Autodesk Fusion 360 part; units mm, degrees
note: some values were not read from the file. Set by a fixed rule: which sketch regions a step uses.
(part 2 of 4)
  dimension "d679" = 4.2
  dimension "d680" = 50.8
  dimension "d681" = 177.3195
  dimension "d682" = 177.3195
  dimension "d683" = 177.3195
  dimension "d684" = 177.3195
  dimension "d685" = 25.4
  dimension "d686" = 25.4
  dimension "d687" = 25.4
  dimension "d688" = 25.4
  dimension "d689" = 4.2
  dimension "d690" = 4.2
  dimension "d691" = 4.2
  dimension "d692" = 4.2
  dimension "d693" = 50.8
  dimension "d697" = 177.3195
  dimension "d698" = 177.3195
  dimension "d699" = 177.3195
  dimension "d700" = 177.3195
  dimension "d701" = 25.4
  dimension "d702" = 25.4
  dimension "d703" = 25.4
  dimension "d704" = 25.4
  dimension "d705" = 4.2
  dimension "d706" = 4.2
  dimension "d707" = 4.2
  dimension "d708" = 4.2
  dimension "d709" = 50.8
  dimension "d710" = 177.3195
  dimension "d711" = 177.3195
  dimension "d712" = 177.3195
  dimension "d713" = 177.3195
  dimension "d714" = 25.4
  dimension "d715" = 25.4
  dimension "d716" = 25.4
  dimension "d717" = 25.4
  dimension "d718" = 4.2
  dimension "d719" = 4.2
  dimension "d720" = 4.2
  dimension "d721" = 4.2
  dimension "d722" = 50.8
  dimension "d723" = 177.3195
  dimension "d724" = 177.3195
  dimension "d725" = 177.3195
  dimension "d726" = 177.3195
  dimension "d727" = 25.4
  dimension "d728" = 25.4
  dimension "d729" = 25.4
  dimension "d730" = 25.4
  dimension "d731" = 4.2
  dimension "d732" = 4.2
  dimension "d733" = 4.2
  dimension "d734" = 4.2
  dimension "d735" = 50.8
  constraint horizontal L6
  constraint vertical L7
  constraint horizontal L5
  constraint vertical L8
  constraint horizontal L0
  constraint perpendicular L0 L27
  constraint horizontal L19
  constraint perpendicular L2 L20
  constraint horizontal L14
  constraint perpendicular L13 L23
  constraint horizontal L4
  constraint perpendicular L29 L30
  constraint perpendicular L0 L12
  constraint tangent A9 L29
  constraint tangent A9 L27
  constraint coincident P14 L0
  constraint coincident P14 L27
  constraint tangent L0 A7
  constraint tangent A7 L27
  constraint tangent L0 A18
  constraint tangent L2 A18
  constraint coincident P13 L2
  constraint coincident P13 L20
  constraint tangent L2 A12
  constraint tangent L20 A12
  constraint coincident P7 L3
  constraint coincident P7 L12
  constraint tangent L3 A15
  constraint tangent L12 A15
  constraint coincident P11 L24
  constraint coincident P11 L12
  constraint tangent L24 A14
  constraint tangent L12 A14
  constraint coincident L14.start L20
  constraint coincident L14.start L24
  constraint tangent L20 A20
  constraint tangent L24 A20
  constraint coincident P8 L30
  constraint coincident P8 L29
  constraint tangent A10 L30
  constraint tangent A10 L29
  constraint coincident L4.start L13
  constraint coincident L4.start L30
  constraint tangent A0 L13
  constraint tangent A0 L30
  constraint coincident P12 L13
  constraint coincident P12 L23
  constraint tangent L13 A17
  constraint tangent L23 A17
  constraint coincident P6 L23
  constraint coincident P6 L3
  constraint tangent A4 L23
  constraint tangent L3 A4
  constraint horizontal L10
  constraint perpendicular L10 L21
  constraint perpendicular L11 L22
  constraint horizontal L16
  constraint perpendicular L25 L26
  constraint perpendicular L9 L17
  constraint perpendicular L10 L18
  constraint tangent L9 A19
  constraint tangent L21 A19
  constraint coincident P14 L10
  constraint coincident P14 L21
  constraint tangent L10 A3
  constraint tangent A3 L21
  constraint tangent L10 A8
  constraint tangent L11 A8
  constraint coincident P13 L11
  constraint coincident P13 L22
  constraint tangent L11 A16
  constraint tangent L22 A16
  constraint coincident P7 L28
  constraint coincident P7 L18
  constraint tangent A22 L28
  constraint tangent L18 A22
  constraint coincident P11 L15
  constraint coincident P11 L18
  constraint tangent L15 A23
  constraint tangent L18 A23
  constraint coincident L14.start L22
  constraint coincident L14.start L15
  constraint tangent A1 L22
  constraint tangent A1 L15
  constraint coincident P8 L17
  constraint coincident P8 L9
  constraint tangent A2 L17
  constraint tangent L9 A2
  constraint tangent A11 L25
  constraint tangent L17 A11
  constraint coincident P12 L25
  constraint coincident P12 L26
  constraint tangent A5 L25
  constraint tangent A5 L26
  constraint coincident P6 L26
  constraint coincident P6 L28
  constraint tangent A13 L26
  constraint tangent A13 L28
  constraint horizontal L1
  constraint coincident L1.start L0
  constraint horizontal L53
  constraint horizontal L36
  constraint horizontal L70
  constraint coincident L48.end L36
  constraint parallel L49 L53
  constraint parallel L38 L71
  constraint collinear L47 L53
  constraint collinear L36 L61
  constraint horizontal L77
  constraint horizontal L76
  constraint horizontal L59
  constraint coincident L54.end L76
  constraint parallel L67 L77
  constraint parallel L55 L64
  constraint collinear L32 L77
  constraint collinear L58 L76
  constraint perpendicular L38 L57
  constraint perpendicular L37 L71
  constraint collinear L44 L71
  constraint collinear L34 L74
  constraint perpendicular L46 L51
  constraint coincident A26.start A31
  constraint perpendicular L39 L66
  constraint concentric A26 A31
  constraint vertical L35
  constraint perpendicular L35 L41
  constraint perpendicular L31 L35
  constraint perpendicular L41 L73
  constraint coincident L65.end L41
  constraint parallel L40 L41
  constraint parallel L33 L73
  constraint parallel L31 L50
  constraint parallel L35 L75
  constraint coincident L40.end A27.centre
  constraint coincident L33.end A25.centre
  constraint coincident A29.centre L50.end
  constraint coincident A24.centre L75.end
  constraint parallel L41 L45
  constraint coincident L31.start L35.start
  constraint coincident L45.end A28
  constraint horizontal L93
  constraint vertical L96
  constraint horizontal L98
  constraint vertical L85
  constraint coincident P15 L85.end
  constraint horizontal L86
  constraint vertical L101
  constraint horizontal L87
  constraint vertical L92
  constraint coincident L87.start A32.centre
  constraint perpendicular L98 L100
  constraint vertical L83
  constraint horizontal L80
  constraint vertical L81
  constraint horizontal L82
  constraint vertical L84
  constraint horizontal L99
  constraint vertical L89
  constraint horizontal L97
  constraint vertical L95
  constraint horizontal L94
  constraint vertical L91
  constraint horizontal L88
  constraint vertical L90
  constraint coincident L89.end L97.start
  constraint coincident L88.start L91.end
  constraint horizontal L102
  constraint vertical L103
  constraint horizontal L104
  constraint vertical L105
  constraint horizontal L112
  constraint perpendicular L112 L125
  constraint horizontal L131
  constraint perpendicular L113 L119
  constraint horizontal L130
  constraint perpendicular L107 L108
  constraint horizontal L128
  constraint perpendicular L106 L116
  constraint perpendicular L112 L120
  constraint tangent L116 A42
  constraint tangent A42 L125
  constraint coincident P26 L112
  constraint coincident P26 L125
  constraint tangent L112 A52
  constraint tangent L125 A52
  constraint tangent A35 L112
  constraint tangent A35 L113
  constraint coincident P28 L113
  constraint coincident P28 L119
  constraint tangent L113 A53
  constraint tangent L119 A53
  constraint coincident P30 L109
  constraint coincident P30 L120
  constraint tangent L109 A49
  constraint tangent L120 A49
  constraint coincident P21 L118
  constraint coincident P21 L120
  constraint tangent L118 A43
  constraint tangent A43 L120
  constraint coincident L122.start L119
  constraint coincident L122.start L118
  constraint tangent L119 A51
  constraint tangent L118 A51
  constraint coincident P22 L106
  constraint coincident P22 L116
  constraint tangent L106 A37
  constraint tangent A37 L116
  constraint coincident L128.start L107
  constraint coincident L128.start L106
  constraint tangent L107 A57
  constraint tangent L106 A57
  constraint coincident P25 L107
  constraint coincident P25 L108
  constraint tangent L107 A41
  constraint tangent L108 A41
  constraint coincident P29 L108
  constraint coincident P29 L109
  constraint tangent L108 A39
  constraint tangent L109 A39
  constraint horizontal L115
  constraint perpendicular L115 L121
  constraint perpendicular L124 L132
  constraint horizontal L122
  constraint perpendicular L114 L129
  constraint perpendicular L110 L127
  constraint perpendicular L115 L123
  constraint tangent L110 A54
  constraint tangent L121 A54
  constraint coincident P26 L115
  constraint coincident P26 L121
  constraint tangent L115 A47
  constraint tangent L121 A47
  constraint tangent L115 A55
  constraint tangent A55 L132
  constraint coincident P28 L132
  constraint coincident P28 L124
  constraint tangent A40 L132
  constraint tangent A40 L124
  constraint coincident P30 L117
  constraint coincident P30 L123
  constraint tangent L117 A45
  constraint tangent A45 L123
  constraint coincident P21 L126
  constraint coincident P21 L123
  constraint tangent A50 L126
  constraint tangent A50 L123
  constraint coincident L122.start L124
  constraint coincident L122.start L126
  constraint tangent A48 L124
  constraint tangent A48 L126
  constraint coincident P22 L127
  constraint coincident P22 L110
  constraint tangent A46 L127
  constraint tangent L110 A46
  constraint tangent A36 L129
  constraint tangent A36 L127
  constraint coincident P25 L129
  constraint coincident P25 L114
  constraint tangent L129 A56
  constraint tangent L114 A56
  constraint coincident P29 L114
  constraint coincident P29 L117
  constraint tangent A38 L114
  constraint tangent A38 L117
  constraint horizontal L111
  constraint coincident L111.start L112
  constraint horizontal L139
  constraint perpendicular L139 L152
  constraint horizontal L158
  constraint perpendicular L140 L146
  constraint horizontal L157
  constraint perpendicular L134 L135
  constraint horizontal L155
  constraint perpendicular L133 L143
  constraint perpendicular L139 L147
  constraint tangent L143 A66
  constraint tangent A66 L152
  constraint coincident P41 L139
  constraint coincident P41 L152
  constraint tangent L139 A76
  constraint tangent L152 A76
  constraint tangent A59 L139
  constraint tangent A59 L140
  constraint coincident P43 L140
  constraint coincident P43 L146
  constraint tangent L140 A77
  constraint tangent L146 A77
  constraint coincident P45 L136
  constraint coincident P45 L147
  constraint tangent L136 A73
  constraint tangent L147 A73
  constraint coincident P36 L145
  constraint coincident P36 L147
  constraint tangent L145 A67
  constraint tangent A67 L147
  constraint coincident L149.start L146
  constraint coincident L149.start L145
  constraint tangent L146 A75
  constraint tangent L145 A75
  constraint coincident P37 L133
  constraint coincident P37 L143
  constraint tangent L133 A61
  constraint tangent A61 L143
  constraint coincident L155.start L134
  constraint coincident L155.start L133
  constraint tangent L134 A81
  constraint tangent L133 A81
  constraint coincident P40 L134
  constraint coincident P40 L135
  constraint tangent L134 A65
  constraint tangent L135 A65
  constraint coincident P44 L135
  constraint coincident P44 L136
  constraint tangent L135 A63
  constraint tangent L136 A63
  constraint horizontal L142
  constraint perpendicular L142 L148
  constraint perpendicular L151 L159
  constraint horizontal L149
  constraint perpendicular L141 L156
  constraint perpendicular L137 L154
  constraint perpendicular L142 L150
  constraint tangent L137 A78
  constraint tangent L148 A78
  constraint coincident P41 L142
  constraint coincident P41 L148
  constraint tangent L142 A71
  constraint tangent L148 A71
  constraint tangent L142 A79
  constraint tangent A79 L159
  constraint coincident P43 L159
  constraint coincident P43 L151
  constraint tangent A64 L159
  constraint tangent A64 L151
  constraint coincident P45 L144
  constraint coincident P45 L150
  constraint tangent L144 A69
  constraint tangent A69 L150
  constraint coincident P36 L153
  constraint coincident P36 L150
  constraint tangent A74 L153
  constraint tangent A74 L150
  constraint coincident L149.start L151
  constraint coincident L149.start L153
  constraint tangent A72 L151
  constraint tangent A72 L153
  constraint coincident P37 L154
  constraint coincident P37 L137
  constraint tangent A70 L154
  constraint tangent L137 A70
  constraint tangent A60 L156
  constraint tangent A60 L154
  constraint coincident P40 L156
  constraint coincident P40 L141
  constraint tangent L156 A80
  constraint tangent L141 A80
  constraint coincident P44 L141
  constraint coincident P44 L144
  constraint tangent A62 L141
  constraint tangent A62 L144
  constraint horizontal L138
  constraint coincident L138.start L139
  constraint horizontal L166
  constraint perpendicular L166 L179
  constraint horizontal L185
  constraint perpendicular L167 L173
  constraint horizontal L184
  constraint perpendicular L161 L162
  constraint horizontal L182
  constraint perpendicular L160 L170
  constraint perpendicular L166 L174
  constraint tangent L170 A90
  constraint tangent A90 L179
  constraint coincident P56 L166
  constraint coincident P56 L179
  constraint tangent L166 A100
  constraint tangent L179 A100
  constraint tangent A83 L166
  constraint tangent A83 L167
  constraint coincident P58 L167
  constraint coincident P58 L173
  constraint tangent L167 A101
  constraint tangent L173 A101
  constraint coincident P60 L163
  constraint coincident P60 L174
  constraint tangent L163 A97
  constraint tangent L174 A97
  constraint coincident P51 L172
  constraint coincident P51 L174
  constraint tangent L172 A91
  constraint tangent A91 L174
  constraint coincident L176.start L173
  constraint coincident L176.start L172
  constraint tangent L173 A99
  constraint tangent L172 A99
  constraint coincident P52 L160
  constraint coincident P52 L170
  constraint tangent L160 A85
  constraint tangent A85 L170
  constraint coincident L182.start L161
  constraint coincident L182.start L160
  constraint tangent L161 A105
  constraint tangent L160 A105
  constraint coincident P55 L161
  constraint coincident P55 L162
  constraint tangent L161 A89
  constraint tangent L162 A89
  constraint coincident P59 L162
  constraint coincident P59 L163
  constraint tangent L162 A87
  constraint tangent L163 A87
  constraint horizontal L169
  constraint perpendicular L169 L175
  constraint perpendicular L178 L186
  constraint horizontal L176
  constraint perpendicular L168 L183
  constraint perpendicular L164 L181
  constraint perpendicular L169 L177
  constraint tangent L164 A102
  constraint tangent L175 A102
  constraint coincident P56 L169
  constraint coincident P56 L175
  constraint tangent L169 A95
  constraint tangent L175 A95
  constraint tangent L169 A103
  constraint tangent A103 L186
  constraint coincident P58 L186
  constraint coincident P58 L178
  constraint tangent A88 L186
  constraint tangent A88 L178
  constraint coincident P60 L171
  constraint coincident P60 L177
  constraint tangent L171 A93
  constraint tangent A93 L177
  constraint coincident P51 L180
  constraint coincident P51 L177
  constraint tangent A98 L180
  constraint tangent A98 L177
  constraint coincident L176.start L178
  constraint coincident L176.start L180
  constraint tangent A96 L178
  constraint tangent A96 L180
  constraint coincident P52 L181
  constraint coincident P52 L164
  constraint tangent A94 L181
  constraint tangent L164 A94
  constraint tangent A84 L183
  constraint tangent A84 L181
  constraint coincident P55 L183
  constraint coincident P55 L168
  constraint tangent L183 A104
  constraint tangent L168 A104
  constraint coincident P59 L168
  constraint coincident P59 L171
  constraint tangent A86 L168
  constraint tangent A86 L171
  constraint horizontal L165
  constraint coincident L165.start L166
  constraint horizontal L188
  constraint vertical L190
  constraint horizontal L187
  constraint vertical L189
  constraint horizontal L205
  constraint vertical L210
  constraint horizontal L207
  constraint vertical L196
  constraint coincident P61 L195.start
  constraint horizontal L195
  constraint vertical L193
  constraint horizontal L203
  constraint vertical L206
  constraint coincident L193.end L203.start
  constraint perpendicular L198 L207
  constraint vertical L209
  constraint horizontal L192
  constraint vertical L199
  constraint horizontal L201
  constraint vertical L204
  constraint horizontal L212
  constraint vertical L211
  constraint horizontal L200
  constraint vertical L197
  constraint horizontal L194
  constraint vertical L191
  constraint horizontal L202
  constraint vertical L208
  constraint coincident L200.start A108.centre
  constraint coincident L191.end A107.centre
  constraint horizontal L227
  constraint vertical L232
  constraint horizontal L229
  constraint vertical L218
  constraint coincident P62 L217.start
  constraint horizontal L217
  constraint vertical L215
  constraint horizontal L225
  constraint vertical L228
  constraint coincident L215.end L225.start
  constraint perpendicular L220 L229
  constraint vertical L231
  constraint horizontal L214
  constraint vertical L221
  constraint horizontal L223
  constraint vertical L226
  constraint horizontal L234
  constraint vertical L233
  constraint horizontal L222
  constraint vertical L219
  constraint horizontal L216
  constraint vertical L213
  constraint horizontal L224
  constraint vertical L230
  constraint coincident L222.start A111.centre
  constraint coincident L213.end A110.centre
  constraint horizontal L249
  constraint vertical L254
  constraint horizontal L251
  constraint vertical L240
  constraint coincident P63 L239.start
  constraint horizontal L239
  constraint vertical L237
  constraint horizontal L247
  constraint vertical L250
  constraint coincident L237.end L247.start
  constraint perpendicular L242 L251
  constraint vertical L253
  constraint horizontal L236
  constraint vertical L243
  constraint horizontal L245
  constraint vertical L248
  constraint horizontal L256
  constraint vertical L255
  constraint horizontal L244
  constraint vertical L241
  constraint horizontal L238
  constraint vertical L235
  constraint horizontal L246
  constraint vertical L252
  constraint coincident L244.start A114.centre
  constraint coincident L235.end A113.centre
  constraint horizontal L261
  constraint vertical L262
  constraint horizontal L263
  constraint vertical L264
  constraint horizontal L268
  constraint vertical L266
  constraint horizontal L265
  constraint vertical L267
  constraint horizontal L273
  constraint horizontal L283
  constraint horizontal L286
  constraint coincident L272.end L283
  constraint parallel L273 L281
  constraint parallel L271 L276
  constraint collinear L273 L282
  constraint collinear L275 L283
  constraint perpendicular L269 L279
  constraint coincident A117.start A116
  constraint perpendicular L277 L287
  constraint concentric A116 A117
  constraint horizontal L288
  constraint vertical L289
  constraint horizontal L290
  constraint vertical L291
  constraint horizontal L292
  constraint vertical L293
  constraint horizontal L294
  constraint vertical L295
  constraint horizontal L296
  constraint vertical L299
  constraint horizontal L297
  constraint vertical L298
  constraint horizontal L300
  constraint vertical L303
  constraint horizontal L301
  constraint vertical L302
  constraint horizontal L315
  constraint vertical L314
  constraint horizontal L312
  constraint vertical L313
  constraint vertical L322
  constraint perpendicular L317 L322
  constraint perpendicular L322 L324
  constraint perpendicular L317 L319
  constraint coincident L65.end L317
  constraint parallel L317 L320
  constraint parallel L318 L319
  constraint parallel L321 L324
  constraint parallel L322 L323
  constraint parallel L317 L325
  constraint coincident L45.end A120
  constraint horizontal L326
  constraint vertical L327
  constraint horizontal L328
  constraint vertical L329
  constraint vertical L336
  constraint perpendicular L330 L336
  constraint perpendicular L333 L336
  constraint perpendicular L330 L338
  constraint coincident L65.end L330
  constraint parallel L330 L343
  constraint parallel L334 L338
  constraint parallel L333 L349
  constraint parallel L336 L348
  constraint parallel L330 L345
  constraint coincident L45.end A126
  constraint vertical L332
  constraint perpendicular L332 L346
  constraint perpendicular L332 L347
  constraint perpendicular L337 L346
  constraint coincident L65.end L346
  constraint parallel L331 L346
  constraint parallel L337 L340
  constraint parallel L339 L347
  constraint parallel L332 L335
  constraint parallel L341 L346
  constraint coincident L45.end A130
  constraint vertical L378
  constraint perpendicular L360 L378
  constraint perpendicular L369 L378
  constraint perpendicular L360 L380
  constraint coincident L65.end L360
  constraint parallel L360 L362
  constraint parallel L380 L382
  constraint parallel L369 L377
  constraint parallel L367 L378
  constraint parallel L360 L361
  constraint coincident L45.end A141
  constraint vertical L386
  constraint perpendicular L364 L386
  constraint perpendicular L379 L386
  constraint perpendicular L364 L368
  constraint coincident L65.end L364
  constraint parallel L351 L364
  constraint parallel L365 L368
  constraint parallel L375 L379
  constraint parallel L386 L387
  constraint parallel L357 L364
  constraint coincident L45.end A136
  constraint vertical L381
  constraint perpendicular L354 L381
  constraint perpendicular L366 L381
  constraint perpendicular L354 L389
  constraint coincident L65.end L354
  constraint parallel L350 L354
  constraint parallel L388 L389
  constraint parallel L366 L370
  constraint parallel L381 L383
  constraint parallel L354 L355
  constraint coincident L45.end A147
  constraint vertical L374
  constraint perpendicular L374 L385
  constraint perpendicular L372 L374
  constraint perpendicular L371 L385
  constraint coincident L65.end L385
  constraint parallel L356 L385
  constraint parallel L371 L384
  constraint parallel L372 L373
  constraint parallel L374 L376
  constraint parallel L352 L385
  constraint coincident L45.end A148
  constraint vertical L446
  constraint perpendicular L431 L446
  constraint perpendicular L441 L446
  constraint perpendicular L431 L434
  constraint coincident L65.end L431
  constraint parallel L398 L431
  constraint parallel L405 L434
  constraint parallel L421 L441
  constraint parallel L446 L448
  constraint parallel L397 L431
  constraint coincident L45.end A174
  constraint vertical L453
  constraint perpendicular L414 L453
  constraint perpendicular L439 L453
  constraint perpendicular L414 L457
  constraint coincident L65.end L414
  constraint parallel L390 L414
  constraint parallel L403 L457
  constraint parallel L420 L439
  constraint parallel L453 L456
  constraint parallel L414 L425
  constraint coincident L45.end A153
  constraint vertical L429
  constraint perpendicular L429 L437
  constraint perpendicular L399 L429
  constraint perpendicular L430 L437
  constraint coincident L65.end L437
  constraint parallel L424 L437
  constraint parallel L412 L430
  constraint parallel L399 L444
  constraint parallel L407 L429
  constraint parallel L437 L461
  constraint coincident L45.end A182
  constraint vertical L406
  constraint perpendicular L406 L413
  constraint perpendicular L406 L447
  constraint perpendicular L413 L433
  constraint coincident L65.end L413
  constraint parallel L413 L459
  constraint parallel L410 L433
  constraint parallel L415 L447
  constraint parallel L406 L455
  constraint parallel L413 L466
  constraint coincident L45.end A175
  constraint vertical L428
  constraint perpendicular L428 L442
  constraint perpendicular L402 L428
  constraint perpendicular L436 L442
  constraint coincident L65.end L442
  constraint parallel L442 L463
  constraint parallel L408 L436
  constraint parallel L402 L416
  constraint parallel L428 L440
  constraint parallel L442 L460
  constraint coincident L45.end A179
  constraint vertical L443
  constraint perpendicular L417 L443
  constraint perpendicular L435 L443
  constraint perpendicular L417 L451
  constraint coincident L65.end L417
  constraint parallel L417 L465
  constraint parallel L409 L451
  constraint parallel L422 L435
  constraint parallel L401 L443
  constraint parallel L417 L464
  constraint coincident L45.end A180
  constraint vertical L438
  constraint perpendicular L438 L445
  constraint perpendicular L438 L450
  constraint perpendicular L445 L454
  constraint coincident L65.end L445
  constraint parallel L445 L462
  constraint parallel L404 L454
  constraint parallel L419 L450
  constraint parallel L427 L438
  constraint parallel L395 L445
  constraint coincident L45.end A173
  constraint vertical L452
  constraint perpendicular L452 L467
  constraint perpendicular L400 L452
  constraint perpendicular L432 L467
  constraint coincident L65.end L467
  constraint parallel L394 L467
  constraint parallel L411 L432
  constraint parallel L400 L418
  constraint parallel L449 L452
  constraint parallel L426 L467
  constraint coincident L45.end A177
  measures "d142" distance of L6.end L6.start
  measures "d143" distance of L6.start L5.end
  measures "d899" distance of P10 P14
  measures "d900" angle of L2 L19
  measures "d901" distance of P10 P13
  measures "d902" distance of L14.start P13
  measures "d903" angle of L14 L24
  measures "d907" distance of P6 P12
  measures "d908" distance of L4.start P12
  measures "d909" angle of L4 L30
  measures "d910" distance of L4.start P8
  measures "d911" distance of P11 P7
  measures "d913" radius of A7
  measures "d914" radius of A18
  measures "d915" radius of A12
  measures "d919" radius of A10
  measures "d920" radius of A0
  measures "d923" distance of P14 P10
  measures "d927" distance of P11 L14.start
  measures "d928" distance of P6 P12
  measures "d933" radius of A19
  measures "d937" radius of A22
  measures "d938" radius of A23
  measures "d939" radius of A1
  measures "d941" radius of A11
  measures "d942" radius of A5
  measures "d943" radius of A13
  measures "d949" diameter of A6
  measures "d950" diameter of A21
  measures "d144" distance of L47.end L36.start
  measures "d147" distance of L56.end L34.end
  measures "d148" distance of L47.end L36.start
  measures "d149" angle of L69 L70
  measures "d150" distance of L34.end L56.end
  measures "d151" distance of L36.end L36.start
  measures "d152" distance of L47.end L47.start
  measures "d153" distance of L43.start L32.end
  measures "d155" distance of L43.end L42.end
  measures "d156" distance of L43.start L32.end
  measures "d157" angle of L59 L79
  measures "d158" distance of L42.end L43.end
  measures "d159" distance of L43.start A26.end
  measures "d160" distance of L32.start L32.end
  measures "d161" distance of L42.end L55.end
  measures "d162" distance of L34.start L57.end
  measures "d163" distance of L37.start L57.end
  measures "d164" distance of L39.start L55.end
  measures "d165" distance of L39.start L46.start
  measures "d166" distance of L39.start L39.end
  measures "d167" distance of L31.start L35.end
  measures "d168" distance of L31.start L40.start
  measures "d169" distance of L31.start L31.end
  measures "d170" distance of L31.start L33.start
  measures "d171" distance of L40.end L40.start
  measures "d172" distance of L33.end L33.start
  measures "d173" distance of L31.end A29.centre
  measures "d174" distance of A24.centre L35.end
  measures "d175" diameter of A27
  measures "d176" diameter of A25
  measures "d177" diameter of A29
  measures "d178" diameter of A24
  measures "d179" distance of L45.end L40.start
  measures "d218" distance of L93.end P15
  measures "d219" distance of L85.start P15
  measures "d220" distance of P15 L86.end
  measures "d221" distance of P15 L87.end
  measures "d222" diameter of A32
  measures "d226" distance of L80.start L80.end
  measures "d227" distance of L80.start L82.end
  measures "d694" diameter of A34
  measures "d695" diameter of A33
  measures "d247" distance of L102.start L102.end
  measures "d248" distance of L102.start L104.end
  measures "d249" distance of P26 P24
  measures "d250" angle of L113 L131
  measures "d251" distance of P28 P24
  measures "d252" distance of L122.start P28
  measures "d253" angle of L118 L130
  measures "d254" distance of P29 P25
  measures "d255" distance of L128.start P25
  measures "d256" angle of L106 L128
  measures "d257" distance of P22 L128.start
  measures "d258" distance of P21 P30
  measures "d259" radius of A52
  measures "d260" radius of A35
  measures "d261" radius of A53
  measures "d262" radius of A37
  measures "d263" radius of A57
  measures "d264" distance of P26 P24
  measures "d265" distance of P21 L122.start
  measures "d266" distance of P25 P29
  measures "d267" radius of A54
  measures "d268" radius of A45
  measures "d269" radius of A50
  measures "d270" radius of A48
  measures "d271" radius of A36
  measures "d272" radius of A56
  measures "d273" radius of A38
  measures "d274" diameter of A58
  measures "d275" diameter of A44
  measures "d276" distance of P41 P39
  measures "d277" angle of L140 L158
  measures "d278" distance of P43 P39
  measures "d279" distance of L149.start P43
  measures "d280" angle of L145 L157
  measures "d281" distance of P44 P40
  measures "d282" distance of L155.start P40
  measures "d283" angle of L133 L155
  measures "d284" distance of P37 L155.start
  measures "d285" distance of P36 P45
  measures "d286" radius of A76
  measures "d287" radius of A59
  measures "d288" radius of A77
  measures "d289" radius of A61
  measures "d290" radius of A81
  measures "d291" distance of P41 P39
  measures "d292" distance of P36 L149.start
  measures "d293" distance of P40 P44
  measures "d294" radius of A78
  measures "d295" radius of A69
  measures "d296" radius of A74
  measures "d297" radius of A72
  measures "d298" radius of A60
  measures "d299" radius of A80
  measures "d300" radius of A62
  measures "d301" diameter of A82
  measures "d302" diameter of A68
  measures "d303" distance of P56 P54
  measures "d304" angle of L167 L185
  measures "d305" distance of P58 P54
  measures "d306" distance of L176.start P58
  measures "d307" angle of L172 L184
  measures "d308" distance of P59 P55
  measures "d309" distance of L182.start P55
  measures "d310" angle of L160 L182
  measures "d311" distance of P52 L182.start
  measures "d312" distance of P51 P60
  measures "d313" radius of A100
  measures "d314" radius of A83
  measures "d315" radius of A101
  measures "d316" radius of A85
  measures "d317" radius of A105
  measures "d318" distance of P56 P54
  measures "d319" distance of P51 L176.start
  measures "d320" distance of P55 P59
  measures "d321" radius of A102
  measures "d322" radius of A93
  measures "d323" radius of A98
  measures "d324" radius of A96
  measures "d325" radius of A84
  measures "d326" radius of A104
  measures "d327" radius of A86
  measures "d328" diameter of A106
  measures "d329" diameter of A92
  measures "d330" distance of L188.start L188.end
  measures "d331" distance of L187.end L188.start
  measures "d332" distance of P61 L205.end
  measures "d333" distance of L194.start P61
  measures "d334" distance of L193.start P61
  measures "d335" distance of P61 L203.end
  measures "d336" diameter of A109
  measures "d337" distance of L192.start L192.end
  measures "d338" distance of L192.start L201.end
  measures "d339" diameter of A108
  measures "d340" diameter of A107
  measures "d341" distance of P62 L227.end
  measures "d342" distance of L216.start P62
  measures "d343" distance of L215.start P62
  measures "d344" distance of P62 L225.end
  measures "d345" diameter of A112
  measures "d346" distance of L214.start L214.end
  measures "d347" distance of L214.start L223.end
  measures "d348" diameter of A111
  measures "d349" diameter of A110
  measures "d350" distance of P63 L249.end
  measures "d351" distance of L238.start P63
  measures "d352" distance of L237.start P63
  measures "d353" distance of P63 L247.end
  measures "d354" diameter of A115
  measures "d355" distance of L236.start L236.end
  measures "d356" distance of L236.start L245.end
  measures "d357" diameter of A114
  measures "d358" diameter of A113
  measures "d359" distance of L258.end L257.start
  measures "d360" distance of L258.end L258.start
  measures "d361" distance of L261.start L261.end
  measures "d362" distance of L261.start L263.end
  measures "d365" distance of L266.start L267.end
  measures "d366" distance of L267.end L265.end
  measures "d367" distance of L270.start L272.start
  measures "d368" distance of L271.end L271.start
  measures "d369" distance of L272.start L270.start
  measures "d370" angle of L280 L286
  measures "d371" distance of L271.end L271.start
  measures "d372" distance of L270.end L270.start
  measures "d373" distance of L272.start L275.start
  measures "d374" distance of L276.end L271.end
  measures "d375" distance of L269.start L276.end
  measures "d376" distance of L269.start L269.end
  measures "d377" distance of L269.start L277.end
  measures "d520" distance of L288.start L288.end
  measures "d521" distance of L288.start L290.end
  measures "d522" distance of L288.start L292.end
  measures "d523" distance of L288.start L294.end
  measures "d524" distance of L296.end L292.end
  measures "d525" distance of L293.end L292.end
  measures "d526" distance of L300.end L296.end
  measures "d527" distance of L297.start L296.end
  measures "d528" distance of L304.end L304.start
  measures "d529" distance of L294.end L304.start
  measures "d530" distance of L308.end L308.start
  measures "d531" distance of L304.start L308.start
  measures "d532" distance of L102.start L102.end
  measures "d533" distance of L102.start L104.end
  measures "d534" distance of L35.end L31.start
  measures "d535" distance of L40.start L31.start
  measures "d536" distance of L31.end L31.start
  measures "d537" distance of L33.start L31.start
  measures "d538" distance of L40.start L40.end
  measures "d539" distance of L33.end L33.start
  measures "d540" distance of L31.end A29.centre
  measures "d541" distance of L35.end A24.centre
  measures "d542" diameter of A121
  measures "d543" diameter of A118
  measures "d544" diameter of A119
  measures "d545" diameter of A122
  measures "d546" distance of L40.start L45.end
  measures "d547" distance of L326.start L326.end
  measures "d548" distance of L326.start L328.end
  measures "d549" distance of L35.end L31.start
  measures "d550" distance of L40.start L31.start
  measures "d551" distance of L31.end L31.start
  measures "d552" distance of L33.start L31.start
  measures "d553" distance of L40.start L40.end
  measures "d554" distance of L33.end L33.start
  measures "d555" distance of L31.end A29.centre
  measures "d556" distance of L35.end A24.centre
  measures "d557" diameter of A127
  measures "d558" diameter of A124
  measures "d559" diameter of A131
  measures "d560" diameter of A132
  measures "d561" distance of L40.start L45.end
  measures "d562" distance of L35.end L31.start
  measures "d563" distance of L40.start L31.start
  measures "d564" distance of L31.end L31.start
  measures "d565" distance of L33.start L31.start
  measures "d566" distance of L40.start L40.end
  measures "d567" distance of L33.start L33.end
  measures "d568" distance of A29.centre L31.end
  measures "d569" distance of L35.end A24.centre
  measures "d570" diameter of A128
  measures "d571" diameter of A129
  measures "d572" diameter of A123
  measures "d573" diameter of A125
  measures "d574" distance of L40.start L45.end
  measures "d575" distance of L35.end L31.start
  measures "d576" distance of L40.start L31.start
  measures "d577" distance of L31.end L31.start
  measures "d578" distance of L33.start L31.start
  measures "d579" distance of L40.start L40.end
  measures "d580" distance of L33.end L33.start
  measures "d581" distance of L31.end A29.centre
  measures "d582" distance of L35.end A24.centre
  measures "d583" diameter of A133
  measures "d584" diameter of A146
  measures "d585" diameter of A140
  measures "d586" diameter of A150
  measures "d587" distance of L40.start L45.end
  measures "d588" distance of L35.end L31.start
  measures "d589" distance of L40.start L31.start
  measures "d590" distance of L31.end L31.start
  measures "d591" distance of L33.start L31.start
  measures "d592" distance of L40.start L40.end
  measures "d593" distance of L33.start L33.end
  measures "d594" distance of A29.centre L31.end
  measures "d595" distance of L35.end A24.centre
  measures "d596" diameter of A135
  measures "d597" diameter of A145
  measures "d598" diameter of A139
  measures "d599" diameter of A144
  measures "d600" distance of L40.start L45.end
  measures "d601" distance of L31.start L35.end
  measures "d602" distance of L31.start L40.start
  measures "d603" distance of L31.start L31.end
  measures "d604" distance of L33.start L31.start
  measures "d605" distance of L40.end L40.start
  measures "d606" distance of L33.start L33.end
  measures "d607" distance of A29.centre L31.end
  measures "d608" distance of A24.centre L35.end
  measures "d609" diameter of A134
  measures "d610" diameter of A152
  measures "d611" diameter of A138
  measures "d612" diameter of A151
  measures "d613" distance of L45.end L40.start
  measures "d614" distance of L31.start L35.end
  measures "d615" distance of L31.start L40.start
  measures "d616" distance of L31.end L31.start
  measures "d617" distance of L31.start L33.start
  measures "d618" distance of L40.end L40.start
  measures "d619" distance of L33.start L33.end
  measures "d620" distance of L31.end A29.centre
  measures "d621" distance of A24.centre L35.end
  measures "d622" diameter of A137
  measures "d623" diameter of A149
  measures "d624" diameter of A143
  measures "d625" diameter of A142
  measures "d626" distance of L45.end L40.start
  measures "d629" distance of L31.start L35.end
  measures "d630" distance of L31.start L40.start
  measures "d631" distance of L31.start L31.end
  measures "d632" distance of L31.start L33.start
  measures "d633" distance of L40.start L40.end
  measures "d634" distance of L33.start L33.end
  measures "d635" distance of L31.end A29.centre
  measures "d636" distance of A24.centre L35.end
  measures "d637" diameter of A190
  measures "d638" diameter of A162
  measures "d639" diameter of A165
  measures "d640" diameter of A160
  measures "d641" distance of L40.start L45.end
  measures "d642" distance of L35.end L31.start
  measures "d643" distance of L31.start L40.start
  measures "d644" distance of L31.end L31.start
  measures "d645" distance of L33.start L31.start
  measures "d646" distance of L40.end L40.start
  measures "d647" distance of L33.end L33.start
  measures "d648" distance of L31.end A29.centre
  measures "d649" distance of L35.end A24.centre
  measures "d650" diameter of A186
  measures "d651" diameter of A157
  measures "d652" diameter of A166
  measures "d653" diameter of A181
  measures "d654" distance of L45.end L40.start
  measures "d655" distance of L31.start L35.end
  measures "d656" distance of L31.start L40.start
  measures "d657" distance of L31.start L31.end
  measures "d658" distance of L31.start L33.start
  measures "d659" distance of L40.start L40.end
  measures "d660" distance of L33.end L33.start
  measures "d661" distance of L31.end A29.centre
  measures "d662" distance of A24.centre L35.end
  measures "d663" diameter of A188
  measures "d664" diameter of A163
  measures "d665" diameter of A171
  measures "d666" diameter of A176
  measures "d667" distance of L45.end L40.start
  measures "d668" distance of L31.start L35.end
  measures "d669" distance of L31.start L40.start
  measures "d670" distance of L31.end L31.start
  measures "d671" distance of L33.start L31.start
  measures "d672" distance of L40.end L40.start
  measures "d673" distance of L33.start L33.end
  measures "d674" distance of L31.end A29.centre
  measures "d675" distance of A24.centre L35.end
  measures "d676" diameter of A192
  measures "d677" diameter of A164
  measures "d678" diameter of A168
  measures "d679" diameter of A159
  measures "d680" distance of L45.end L40.start
  measures "d681" distance of L35.end L31.start
  measures "d682" distance of L40.start L31.start
  measures "d683" distance of L31.end L31.start
  measures "d684" distance of L33.start L31.start
  measures "d685" distance of L40.end L40.start
  measures "d686" distance of L33.start L33.end
  measures "d687" distance of A29.centre L31.end
  measures "d688" distance of L35.end A24.centre
  measures "d689" diameter of A191
  measures "d690" diameter of A155
  measures "d691" diameter of A170
  measures "d692" diameter of A178
  measures "d693" distance of L40.start L45.end
  measures "d697" distance of L35.end L31.start
  measures "d698" distance of L40.start L31.start
  measures "d699" distance of L31.end L31.start
  measures "d700" distance of L33.start L31.start
  measures "d701" distance of L40.end L40.start
  measures "d702" distance of L33.end L33.start
  measures "d703" distance of A29.centre L31.end
  measures "d704" distance of A24.centre L35.end
  measures "d705" diameter of A187
  measures "d706" diameter of A156
  measures "d707" diameter of A167
  measures "d708" diameter of A183
  measures "d709" distance of L45.end L40.start
  measures "d710" distance of L31.start L35.end
  measures "d711" distance of L31.start L40.start
  measures "d712" distance of L31.start L31.end
  measures "d713" distance of L31.start L33.start
  measures "d714" distance of L40.end L40.start
  measures "d715" distance of L33.start L33.end
  measures "d716" distance of A29.centre L31.end
  measures "d717" distance of L35.end A24.centre
  measures "d718" diameter of A185
  measures "d719" diameter of A154
  measures "d720" diameter of A172
  measures "d721" diameter of A184
  measures "d722" distance of L45.end L40.start
  measures "d723" distance of L35.end L31.start
  measures "d724" distance of L40.start L31.start
  measures "d725" distance of L31.end L31.start
  measures "d726" distance of L33.start L31.start
  measures "d727" distance of L40.start L40.end
  measures "d728" distance of L33.start L33.end
  measures "d729" distance of A29.centre L31.end
  measures "d730" distance of L35.end A24.centre
  measures "d731" diameter of A189
  measures "d732" diameter of A161
  measures "d733" diameter of A169
  measures "d734" diameter of A158
  measures "d735" distance of L40.start L45.end